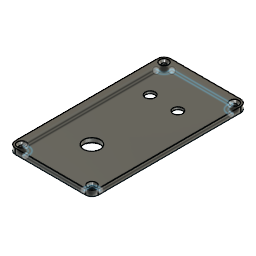
top_shield (Autodesk Fusion 360 design; units mm, degrees)
part number: 2025-12-11-08-38-01-153
Autodesk Fusion 360 part; units mm, degrees
sketch "Esquisse1" plane through (0, 0, 0) normal (0, 0, 1) x (1, 0, 0)
  line L0 (0, 0) -> (60, 0)
  line L1 (60, 0) -> (60, -112)
  line L2 (60, -112) -> (0, -112)
  line L3 (0, -112) -> (0, 0)
  dimension "d1" = 60
  dimension "d2" = 112
  constraint horizontal L0
  constraint vertical L1
  constraint horizontal L2
  constraint vertical L3
  constraint coincident L0.start L3.end
  measures "d1" distance of L0.start L0.end
  measures "d2" distance of L0.start L2.end
extrude "Extrusion1" add sketch "Esquisse1" along normal blind 4
sketch "Esquisse2" plane through (0, 0, 4) normal (0, 0, 1) x (-1, 0, 0)
  line L0 (0, 112) -> (-60, 112)
  line L1 (-60, 112) -> (-60, 0)
  line L2 (-60, 0) -> (0, 0)
  line L3 (0, 0) -> (0, 112)
  circle A0 centre (-4.6, 4.6) radius 1.6
  circle A1 centre (-4.6, 4.6) radius 1.6
  circle A2 centre (-55.4, 4.6) radius 1.6
  circle A3 centre (-4.6, 107.4) radius 1.6
  circle A4 centre (-55.4, 107.4) radius 1.6
  dimension "d5" = 3.2
  dimension "d6" = 4.6
  dimension "d7" = 4.6
  dimension "d8" = 3.2
  dimension "d9" = 3.2
  dimension "d10" = 4.6
  dimension "d11" = 4.6
  dimension "d12" = 3.2
  dimension "d13" = 4.6
  dimension "d14" = 4.6
  dimension "d15" = 3.2
  dimension "d16" = 4.6
  dimension "d17" = 4.6
  measures "d5" diameter of A0
  measures "d6" distance of L3 A0.centre
  measures "d7" distance of L2 A0.centre
  measures "d8" diameter of A1
  measures "d9" diameter of A2
  measures "d10" distance of L1 A2.centre
  measures "d11" distance of L2 A2.centre
  measures "d12" diameter of A3
  measures "d13" distance of L0 A3.centre
  measures "d14" distance of L3 A3.centre
  measures "d15" diameter of A4
  measures "d16" distance of L1 A4.centre
  measures "d17" distance of L0 A4.centre
hole "Perçage1" at (4.6, -4.6, 4) at (55.4, -4.6, 4) at (55.4, -107.4, 4) at (4.6, -107.4, 4) direction (0, 0, -1) diameter 3.2 depth 25 tip angle 118 countersink diameter 6.3 countersink angle 90
fillet "Congé1" radius 4.6 4 edges at (0, 0, 2) (60, 0, 2) (60, -112, 2) (0, -112, 2)
sketch "Esquisse3" plane through (0, 0, 0) normal (0, 0, -1) x (1, 0, 0)
  circle A0 centre (55.4, 107.4) radius 1.6
  circle A1 centre (4.6, 4.6) radius 1.6
  circle A2 centre (55.4, 4.6) radius 1.6
  circle A3 centre (4.6, 107.4) radius 1.6
  arc A4 (4.6, 112) -> (0, 107.4) centre (4.6, 107.4) ccw
  line L0 (0, 107.4) -> (0, 4.6)
  arc A5 (0, 4.6) -> (4.6, 0) centre (4.6, 4.6) ccw
  line L1 (4.6, 0) -> (55.4, 0)
  arc A6 (55.4, 0) -> (60, 4.6) centre (55.4, 4.6) ccw
  line L2 (60, 4.6) -> (60, 107.4)
  arc A7 (60, 107.4) -> (55.4, 112) centre (55.4, 107.4) ccw
  line L3 (55.4, 112) -> (4.6, 112)
  line L4 (8.9, 110) -> (51.6, 110)
  line L5 (2, 8.7) -> (2, 103.1)
  line L6 (52.1, 107.4) -> (52.1, 109.5)
  arc A8 (52.1, 107.4) -> (55.4467, 104.1003) centre (55.4, 107.4) ccw
  line L7 (55.3533, 104.1003) -> (57.5, 104.1003)
  arc A9 (52.1, 109.5) -> (51.6, 110) centre (51.6, 109.5) ccw
  arc A10 (58, 103.6003) -> (57.5, 104.1003) centre (57.5, 103.6003) ccw
  line L8 (7.9, 109) -> (7.9, 107.4)
  line L9 (3, 104.1) -> (4.6, 104.1)
  arc A11 (4.6, 104.1) -> (7.9, 107.4) centre (4.6, 107.4) ccw
  line L10 (3, 7.7) -> (4.6, 7.7)
  line L11 (7.7, 3) -> (7.7, 4.6)
  arc A12 (7.7, 4.6) -> (4.6, 7.7) centre (4.6, 4.6) ccw
  line L12 (57, 7.7) -> (55.4, 7.7)
  line L13 (52.3, 3) -> (52.3, 4.6)
  arc A13 (55.4, 7.7) -> (52.3, 4.6) centre (55.4, 4.6) ccw
  line L14 (58, 103.6003) -> (58, 8.7)
  line L15 (51.3, 2) -> (8.7, 2)
  arc A14 (8.9, 110) -> (7.9, 109) centre (8.9, 109) ccw
  arc A15 (3, 104.1) -> (2, 103.1) centre (3, 103.1) ccw
  arc A16 (2, 8.7) -> (3, 7.7) centre (3, 8.7) ccw
  arc A17 (7.7, 3) -> (8.7, 2) centre (8.7, 3) ccw
  arc A18 (51.3, 2) -> (52.3, 3) centre (51.3, 3) ccw
  arc A19 (57, 7.7) -> (58, 8.7) centre (57, 8.7) ccw
  line L16 (55.4592, 102.1003) -> (56, 102.1003)
  line L17 (56, 102.1003) -> (56, 9.7)
  line L18 (56, 9.7) -> (55.4, 9.7)
  arc A20 (55.4, 9.7) -> (50.3, 4.6) centre (55.4, 4.6) ccw
  line L19 (50.3, 4) -> (50.3, 4.6)
  line L20 (50.3, 4) -> (9.7, 4)
  line L21 (9.7, 4) -> (9.7, 4.6)
  arc A21 (9.7, 4.6) -> (4.6, 9.7) centre (4.6, 4.6) ccw
  line L22 (4, 9.7) -> (4.6, 9.7)
  line L23 (4, 9.7) -> (4, 102.1)
  line L24 (4, 102.1) -> (4.6, 102.1)
  arc A22 (4.6, 102.1) -> (9.9, 107.4) centre (4.6, 107.4) ccw
  line L25 (9.9, 108) -> (9.9, 107.4)
  line L26 (9.9, 108) -> (50.1, 108)
  line L27 (50.1, 107.4) -> (50.1, 108)
  arc A23 (50.1, 107.4) -> (55.4592, 102.1003) centre (55.4, 107.4) ccw
  dimension "d25" = 2
  dimension "d27" = 2
  dimension "d28" = 2
  dimension "d30" = 0.5
  dimension "d31" = 0.5
  dimension "d36" = 1
  dimension "d37" = 2
  constraint horizontal L4
  constraint vertical L14
  constraint vertical L5
  constraint concentric A0 A8
  constraint perpendicular L4 L6
  constraint coincident A8 L7.start
  constraint horizontal L7
  constraint coincident L7 A8.end
  constraint tangent L4 A9
  constraint tangent L6 A9
  constraint tangent L7 A10
  constraint tangent A10 L14
  constraint concentric A3 A11
  constraint perpendicular L4 L8
  constraint tangent L8 A11
  constraint perpendicular L5 L9
  constraint tangent L9 A11
  constraint perpendicular L5 L10
  constraint concentric A1 A12
  constraint tangent L10 A12
  constraint tangent L11 A12
  constraint concentric A2 A13
  constraint perpendicular L12 L14
  constraint tangent L13 A13
  constraint tangent L12 A13
  constraint tangent L8 A14
  constraint tangent L4 A14
  constraint tangent L9 A15
  constraint tangent L5 A15
  constraint equal A14 A15
  constraint tangent L10 A16
  constraint tangent L5 A16
  constraint equal A14 A16
  constraint tangent L11 A17
  constraint tangent L15 A17
  constraint equal A14 A17
  constraint tangent L13 A18
  constraint tangent L15 A18
  constraint equal A14 A18
  constraint tangent L12 A19
  constraint tangent L14 A19
  constraint equal A14 A19
  measures "d25" distance of L3 L4
  measures "d27" distance of L2 L14
  measures "d28" distance of L0 L5
  measures "d30" radius of A9
  measures "d31" radius of A10
  measures "d36" radius of A14
sketch "Esquisse5" plane through (0, 0, 0) normal (0, 0, -1) x (1, 0, 0)
  circle A0 centre (30, 82.0769) radius 6
  dimension "d42" = 12
  measures "d42" diameter of A0
extrude "Extrusion4" cut sketch "Esquisse5" against normal blind 9
chamfer "Chanfrein1" distance 1 angle 45 1 edges at (24.406, -84.2466, 0)
extrude "Extrusion2" add sketch "Esquisse3" along normal blind 1.5 contours L4 L5 L6 A8 L7 A9 A10 L8 L9 A11 L10 L11 A12 L12 L13 A13 L14 L15 A14 A15 A16 A17 A18 A19
extrude "Extrusion3" cut 1 faces at (29.8256, -30.6684, 0) along direction (0, 0, 1) blind 2.2
sketch "Esquisse6" plane through (0, 0, 4) normal (0, 0, 1) x (-1, 0, 0)
  circle A0 centre (-30, 82.0769) radius 6
  arc A1 (0, 107.4) -> (-4.6, 112) centre (-4.6, 107.4) ccw
  line L0 (-4.6, 112) -> (-55.4, 112)
  arc A2 (-55.4, 112) -> (-60, 107.4) centre (-55.4, 107.4) ccw
  line L1 (-60, 107.4) -> (-60, 4.6)
  arc A3 (-60, 4.6) -> (-55.4, 0) centre (-55.4, 4.6) ccw
  line L2 (-55.4, 0) -> (-4.6, 0)
  arc A4 (-4.6, 0) -> (0, 4.6) centre (-4.6, 4.6) ccw
  line L3 (0, 4.6) -> (0, 107.4)
  circle A5 centre (-55.4, 107.4) radius 3.15
  circle A6 centre (-4.6, 4.6) radius 3.15
  circle A7 centre (-55.4, 4.6) radius 3.15
  circle A8 centre (-4.6, 107.4) radius 3.15
  circle A9 centre (-20, 30) radius 3.5
  circle A10 centre (-40, 30) radius 3.5
  dimension "d52" = 7
  dimension "d53" = 30
  dimension "d54" = 7
  dimension "d55" = 30
  dimension "d56" = 20
  dimension "d57" = 20
  measures "d52" diameter of A9
  measures "d53" distance of L2 A9.centre
  measures "d54" diameter of A10
  measures "d55" distance of L2 A10.centre
  measures "d56" distance of L1 A10.centre
  measures "d57" distance of L3 A9.centre
extrude "Extrusion5" cut sketch "Esquisse6" against normal blind 20 contours A9 | A10
equation "d6 = 3 mm + ( 3.2 / 2 ) * 1 mm"
